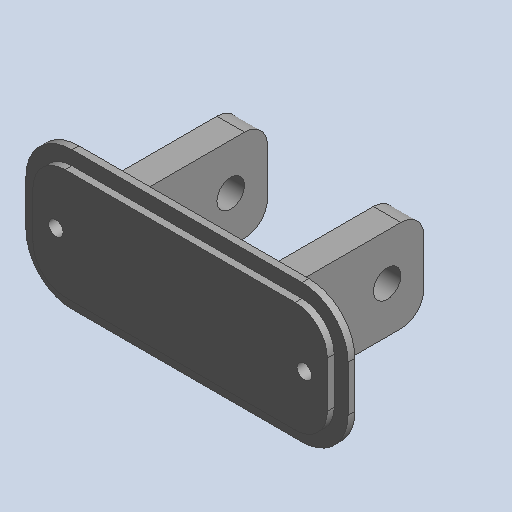
# Autodesk Inventor part: sensor_cover_ultrasonic_2
Saved by Autodesk Inventor 2026 (Build 300175050, 175E)
## iProperties
Part Number: sensor_cover_ultrasonic_2
Material: Generic
Document SubType Name: Modeling
Designer: Kartik
Mass: 11.9458 g
Surface Area: 77.1536 cm^2
Volume: 11.9458 cm^3
Density: 1 g/cm^3
Appearance: Default
Author: Kartik
Autodesk Inventor part; units mm, degrees
ref_plane "YZ Plane" through (0, 0, 0) normal (1, 0, 0) x (0, 1, 0)
ref_plane "XZ Plane" through (0, 0, 0) normal (0, 1, 0) x (-1, 0, 0)
ref_plane "XY Plane" through (0, 0, 0) normal (0, 0, 1) x (1, 0, 0)
sketch "Sketch1" plane through (0, 0, 0) normal (0, 0, 1) x (1, 0, 0)
  line L0 (-35, 15) -> (35, 15)
  line L1 (35, 15) -> (35, -15)
  line L2 (35, -15) -> (-35, -15)
  line L3 (-35, -15) -> (-35, 15)
  point P0 (0, 0)
  dimension "d0" = 70
  dimension "d1" = 30
  dimension "d7" = 35
  dimension "d8" = 15
  constraints: 8 end point, 2 parallel, 1 horizontal, 1 perpendicular
  measures "d0" distance of L0.start L0.end
  measures "d1" distance of L2.end L0.start
  measures "d7" distance from line of L3 point (0, 0)
  measures "d8" distance from line of L0 point (0, 0)
extrude "Extrusion1" add sketch "Sketch1" along normal blind 3
fillet "Fillet1" radius 10 4 edges at (-35, 15, 1.5) (-35, -15, 1.5) (35, -15, 1.5) (35, 15, 1.5)
sketch "Sketch6" plane through (0, 0, 3) normal (0, 0, 1) x (1, 0, 0)
  arc A0 (35, 5) -> (25, 15) centre (25, 5) ccw projected
  line L0 (25, 15) -> (-25, 15) projected
  arc A1 (-25, 15) -> (-35, 5) centre (-25, 5) ccw projected
  line L1 (-35, 5) -> (-35, -5) projected
  arc A2 (-35, -5) -> (-25, -15) centre (-25, -5) ccw projected
  line L2 (-25, -15) -> (25, -15) projected
  arc A3 (25, -15) -> (35, -5) centre (25, -5) ccw projected
  line L3 (35, -5) -> (35, 5) projected
  arc A4 (-25, 12) -> (-32, 5) centre (-25, 5) ccw
  line L4 (-25, 12) -> (25, 12)
  arc A5 (32, 5) -> (25, 12) centre (25, 5) ccw
  line L5 (32, 5) -> (32, -5)
  arc A6 (25, -12) -> (32, -5) centre (25, -5) ccw
  line L6 (25, -12) -> (-25, -12)
  arc A7 (-32, -5) -> (-25, -12) centre (-25, -5) ccw
  line L7 (-32, -5) -> (-32, 5)
  point P0 (0, 0)
  dimension "d43" = 3
  constraints: 8 end point, 8 point on circle, 4 centre point, 7 other
  measures "d43" radial gap between concentric circles of A1 A4
extrude "Extrusion5" cut sketch "Sketch6" against normal blind 1.5
sketch "Sketch7" plane through (0, 0, 3) normal (0, 0, 1) x (1, 0, 0)
  line L0 (-35, -5) -> (-35, 5) projected
  line L1 (35, 5) -> (35, -5) projected
  circle A0 centre (-27, 0) radius 1.6
  circle A1 centre (27, 0) radius 1.6
  point P0 (0, 0)
  point P1 (-35, 0)
  dimension "d46" = 3.2
  dimension "d47" = 8
  dimension "d48" = 3.2
  dimension "d49" = 8
  constraints: 2 centre point, 1 midpoint
  measures "d46" diameter of A0
  measures "d47" distance of point (-35, 0) A0.centre
  measures "d48" diameter of A1
  measures "d49" distance from line of L1 A1.centre
extrude "Extrusion6" cut sketch "Sketch7" against normal through all
sketch "Sketch8" plane through (0, 0, 0) normal (0, 0, -1) x (-1, 0, 0)
  line L0 (-20, 10.5653) -> (-14, 10.5653)
  line L1 (-14, 10.5653) -> (-14, -9.4347)
  line L2 (-14, -9.4347) -> (-20, -9.4347)
  line L3 (-20, -9.4347) -> (-20, 10.5653)
  line L4 (14, 10.5653) -> (20, 10.5653)
  line L5 (20, 10.5653) -> (20, -9.4347)
  line L6 (20, -9.4347) -> (14, -9.4347)
  line L7 (14, -9.4347) -> (14, 10.5653)
  line L8 (-35, -5) -> (-35, 5) projected
  line L9 (35, 5) -> (35, -5) projected
  point P0 (0, 0)
  point P1 (-35, 0)
  dimension "d52" = 20
  dimension "d53" = 6
  dimension "d54" = 6
  dimension "d55" = 15
  dimension "d56" = 15
  constraints: 16 end point, 4 parallel, 2 horizontal, 2 perpendicular, 2 point on line, 1 midpoint
  measures "d52" distance of L2.end L0.start
  measures "d53" distance of L0.start L0.end
  measures "d54" distance of L4.start L4.end
  measures "d55" distance from line of point (-35, 0) L3
  measures "d56" distance between parallel lines of L9 L5
extrude "Extrusion7" add sketch "Sketch8" along normal blind 30
sketch "Sketch9" plane through (20, -9.4347, 0) normal (1, 0, 0) x (0, 0, -1)
  circle A0 centre (22, 10) radius 3
  line L0 (0, 0) -> (30, 0) projected
  line L1 (30, 20) -> (30, 0) projected
  point P0 (0, 9.4347)
  dimension "d59" = 6
  dimension "d60" = 10
  dimension "d61" = 8
  constraints: 1 centre point
  measures "d59" diameter of A0
  measures "d60" distance from line of L0 A0.centre
  measures "d61" distance from line of L1 A0.centre
extrude "Extrusion8" cut sketch "Sketch9" against normal through all
fillet "Fillet2" radius 5 4 edges at (17, -9.4347, -30) (17, 10.5653, -30) (-17, 10.5653, -30) (-17, -9.4347, -30)
equation "\"d7\" = 0.5 * d0"
equation "\"d8\" = 0.5 * d1"
body "Solid1"
